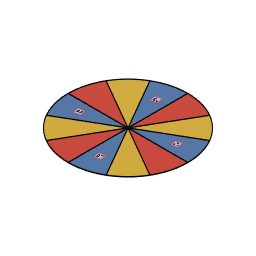
Parachute (Autodesk Fusion 360 design; units mm, degrees)
Autodesk Fusion 360 part; units mm, degrees
sketch "Schizzo1" plane through (0, 0, 0) normal (0, 0, 1) x (1, 0, 0)
  circle A0 centre (0, 0) radius 1500
  line L0 (0, 0) -> (0, 1500)
  line L1 (0, 0) -> (-750, 1299.0381)
  line L2 (0, 0) -> (-1299.0381, 750)
  line L3 (0, 0) -> (-1500, 0)
  line L4 (0, 0) -> (-1299.0381, -750)
  line L5 (0, 0) -> (-750, -1299.0381)
  line L6 (0, 0) -> (0, -1500)
  line L7 (0, 0) -> (750, -1299.0381)
  line L8 (0, 0) -> (1299.0381, -750)
  line L9 (0, 0) -> (1500, 0)
  line L10 (0, 0) -> (1299.0381, 750)
  line L11 (0, 0) -> (750, 1299.0381)
  dimension "d1" = 3000
  dimension "d3" = 360
  constraint coincident A0.centre L0.start
  constraint coincident A0 L0.end
  constraint vertical L0
  measures "d1" diameter of A0
extrude "Estrusione1" add sketch "Schizzo1" along normal blind 10 contours A0 L0 L11 makes body 1
pattern_circular "Serie C1" count 12 over 360 about axis through (0, 0, 1.75) along (0, 0, 1) of bodies 1 makes body 2 at (-441.3417, 894.9525, 0) makes body 3 at (-829.6894, 554.3807, 0) makes body 4 at (-995.7224, 65.2631, 0) makes body 5 at (-894.9525, -441.3417, 0) makes body 6 at (-554.3807, -829.6894, 0) makes body 7 at (-65.2631, -995.7224, 0) makes body 8 at (441.3417, -894.9525, 0) makes body 9 at (829.6894, -554.3807, 0) makes body 10 at (995.7224, -65.2631, 0) makes body 11 at (894.9525, 441.3417, 0) makes body 12 at (554.3807, 829.6894, 0)
sketch "Schizzo2" plane through (0, 0, 10) normal (0, 0, 1) x (-1, 0, 0)
  line L0 (0, 0) -> (0, -1500)
  arc A0 (0, -1500) -> (750, -1299.0381) centre (0, 0) ccw
  line L1 (750, -1299.0381) -> (0, 0)
  line L2 (388.2286, -1448.8887) -> (0, 0) construction
  line L3 (205.786, -1057.7817) -> (350.6749, -1018.9588)
  line L4 (350.6749, -1018.9588) -> (311.8521, -874.07)
  line L5 (311.8521, -874.07) -> (166.9632, -912.8928)
  line L6 (166.9632, -912.8928) -> (205.786, -1057.7817)
  line L7 (205.786, -1057.7817) -> (311.8521, -874.07) construction
  line L8 (350.6749, -1018.9588) -> (166.9632, -912.8928) construction
  line L9 (874.07, 311.8521) -> (912.8928, 166.9632)
  line L10 (1018.9588, 350.6749) -> (874.07, 311.8521)
  line L11 (1057.7817, 205.786) -> (1018.9588, 350.6749)
  line L12 (912.8928, 166.9632) -> (1057.7817, 205.786)
  line L13 (-311.8521, 874.07) -> (-166.9632, 912.8928)
  line L14 (-350.6749, 1018.9588) -> (-311.8521, 874.07)
  line L15 (-205.786, 1057.7817) -> (-350.6749, 1018.9588)
  line L16 (-166.9632, 912.8928) -> (-205.786, 1057.7817)
  line L17 (-874.07, -311.8521) -> (-912.8928, -166.9632)
  line L18 (-1018.9588, -350.6749) -> (-874.07, -311.8521)
  line L19 (-1057.7817, -205.786) -> (-1018.9588, -350.6749)
  line L20 (-912.8928, -166.9632) -> (-1057.7817, -205.786)
  point P0 (258.819, -965.9258)
  dimension "d8" = 500
  dimension "d9" = 150
  dimension "d10" = 150
  dimension "d12" = 360
  constraint midpoint A0 L2.start
  constraint coincident L0.start A0.centre
  constraint perpendicular L3 L4
  constraint parallel L3 L5
  constraint parallel L4 L6
  constraint coincident L7 P0
  constraint coincident L8 P0
  constraint coincident L2 P0
  constraint parallel L2 L6
  measures "d8" distance of L2.start P0
  measures "d9" distance of L3.start L3.end
  measures "d10" distance of L3.start L5.end
component "Component" placed x (1, 0, 0) y (0, 1, 0) z (0, 0, 1) at (0, 0, 0)
